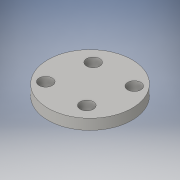
# Autodesk Inventor part: motor_mount
Saved by Autodesk Inventor 2016 (Build 200138000, 138)
## iProperties
Created: 2016-03-06
Part Number: motor_mount
Material: Generic
Document SubType Name: Modeling
Designer: dimas
Density: 1 g/cm^3
Appearance: Default
Author: dimas
Autodesk Inventor part; units mm, degrees
ref_plane "YZ Plane" through (0, 0, 0) normal (1, 0, 0) x (0, 1, 0)
ref_plane "XZ Plane" through (0, 0, 0) normal (0, 1, 0) x (-1, 0, 0)
ref_plane "XY Plane" through (0, 0, 0) normal (0, 0, 1) x (1, 0, 0)
sketch "Sketch1" plane through (0, 0, 0) normal (0, 1, 0) x (-1, 0, 0)
  circle A0 centre (0, 0) radius 9.5
  circle A1 centre (0, 0) radius 8
  circle A2 centre (0, 0) radius 12.7
  dimension "d0" = 19
  dimension "d1" = 16
  dimension "d2" = 25.4
  constraints: 3 centre point, 3 coincident
  measures "d0" diameter of A0
  measures "d1" diameter of A1
  measures "d2" diameter of A2
extrude "Extrusion1" add sketch "Sketch1" along normal blind 3.175 contours A0 | A1 | A2
sketch "Sketch2" plane through (0, 3.175, 0) normal (0, 1, 0) x (1, 0, 0)
  circle A0 centre (0, 0) radius 8
  circle A1 centre (0, 0) radius 9.5
  line L0 (0, 0) -> (0, -6.1214)
  line L1 (0, -6.1214) -> (5.1506, -6.1214)
  line L2 (0, -6.1214) -> (-7.2649, -6.1214)
  line L3 (0, 0) -> (0, 6.1214)
  line L4 (0, 6.1214) -> (-5.1506, 6.1214)
  line L5 (0, 6.1214) -> (7.2649, 6.1214)
  dimension "d5" = 16
  dimension "d6" = 19
  dimension "d7" = 6.1214
  dimension "d8" = 6.1214
  constraints: 12 end point, 4 point on circle, 2 centre point, 2 coincident, 2 point on line, 2 vertical, 1 horizontal, 1 perpendicular
  measures "d5" diameter of A0
  measures "d6" diameter of A1
  measures "d7" distance of L0.start L0.end
  measures "d8" distance of L0.start L3.end
hole "Hole1" at (-7.2649, 3.175, 6.1214) at (-5.1506, 3.175, -6.1214) at (7.2649, 3.175, -6.1214) at (5.1506, 3.175, 6.1214) direction (0, -1, 0) diameter 4 end through all
body "Solid1"
